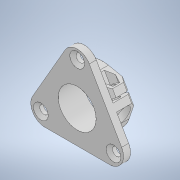
# Autodesk Inventor part: Motor Mount Insert
Saved by Autodesk Inventor 2022 (Build 260153000, 153)
## iProperties
Created: 2022-08-19
Part Number: Motor Mount Insert
Material: Generic
Document SubType Name: Modeling
Designer: Nick
Density: 1.32599 g/cm^3
Appearance: Default
Mass: 5.34 g
Surface Area: 34.9008 cm^2
Volume: 4.02719 cm^3
Author: Nick
Autodesk Inventor part; units mm, degrees
ref_plane "YZ Plane" through (0, 0, 0) normal (1, 0, 0) x (0, 1, 0)
ref_plane "XZ Plane" through (0, 0, 0) normal (0, 1, 0) x (-1, 0, 0)
ref_plane "XY Plane" through (0, 0, 0) normal (0, 0, 1) x (1, 0, 0)
sketch "Sketch1" plane through (0, 0, 0) normal (0, 0, 1) x (1, 0, 0)
  circle A0 centre (0, 16) radius 2
  circle A1 centre (-13.8564, -8) radius 2
  circle A2 centre (13.8564, -8) radius 2
  line L0 (0, 28) -> (24.2487, -14)
  line L1 (24.2487, -14) -> (-24.2487, -14)
  line L2 (-24.2487, -14) -> (0, 28)
  circle A3 centre (0, 0) radius 8.1
  line L3 (0, 16) -> (13.8564, -8) construction
  line L4 (13.8564, -8) -> (-13.8564, -8) construction
  line L5 (-13.8564, -8) -> (0, 16) construction
  dimension "d0" = 16.2
  dimension "d1" = 4
  dimension "d2" = 4
  dimension "d3" = 4
  dimension "d4" = 16
  dimension "d5" = 6
  constraints: 12 end point, 6 coincident, 4 centre point, 2 horizontal, 14 other
  measures "d0" diameter of A3
  measures "d1" diameter of A2
  measures "d2" diameter of A1
  measures "d3" diameter of A0
  measures "d4" distance of point (0, 0) A0.centre
  measures "d5" distance between parallel lines of L0 L3
extrude "Extrusion1" add sketch "Sketch1" along normal blind 3 contours A0 | A1 | A2 | L0 L1 L2
fillet "Fillet1" radius 6 3 edges at (0, 28, 1.5) (24.2487, -14, 1.5) (-24.2487, -14, 1.5)
sketch "Sketch2" plane through (0, 0, 0) normal (0, 0, -1) x (-1, 0, 0)
  circle A0 centre (0, 0) radius 8.1 projected
  arc A1 (13.8564, -14) -> (19.0526, -5) centre (13.8564, -8) ccw projected
  line L0 (5.1962, 19) -> (19.0526, -5) projected
  arc A2 (5.1962, 19) -> (-5.1962, 19) centre (0, 16) ccw projected
  line L1 (-19.0526, -5) -> (-5.1962, 19) projected
  arc A3 (-19.0526, -5) -> (-13.8564, -14) centre (-13.8564, -8) ccw projected
  line L2 (13.8564, -14) -> (-13.8564, -14) projected
  circle A4 centre (0, 0) radius 11.9
  line L3 (-10.5557, 5.517) -> (-10.0557, 6.383)
  line L4 (-10.0557, 6.383) -> (-6.7514, 4.4753)
  line L5 (-6.7514, 4.4753) -> (-7.2514, 3.6093)
  line L6 (-7.2514, 3.6093) -> (-10.5557, 5.517)
  line L7 (0, 0) -> (-7.0014, 4.0423) construction
  circle A5 centre (0, 0) radius 8.1 construction
  line L8 (-10.0557, 6.383) -> (-11.8744, 7.433)
  line L9 (-10.5557, 5.517) -> (-12.3744, 6.567)
  line L10 (-19.0526, -5) -> (-5.1962, 19) projected
  line L11 (-13.8744, 3.9689) -> (-11.286, -3.7732)
  line L12 (-10.3744, 10.0311) -> (-2.3753, 11.6605)
  point P0 (-10.3744, 10.0311)
  point P1 (-7.2514, 3.6093)
  point P2 (-12.3744, 6.567)
  point P3 (-13.8744, 3.9689)
  dimension "d9" = 3.8
  dimension "d10" = 1
  dimension "d11" = 3
  dimension "d12" = 3
  constraints: 18 end point, 5 perpendicular, 4 point on line, 3 point on circle, 3 tangent, 2 parallel, 1 centre point, 1 midpoint, 2 other
  measures "d10" distance between parallel lines of L6 L4
  measures "d11" distance of L9.end L11.start
  measures "d12" distance of L12.start L8.end
extrude "Extrusion2" add sketch "Sketch2" along normal blind 8 contours A0 L4 A4 L6 | L4 L8 L1 L12 A4 | A4 L11 L1 L9 L6 picked at (10.5244, -0.9233)
sketch "Sketch3" plane through (6.7514, 4.4753, -8) normal (0.5, -0.8660254, 0) x (0.8660254, 0.5, 0)
  circle A0 centre (2.9577, 4) radius 1.5
  line L0 (0.4577, 5.4434) -> (2.9577, 6.8868)
  line L1 (2.9577, 6.8868) -> (5.4577, 5.4434)
  line L2 (5.4577, 5.4434) -> (5.4577, 2.5566)
  line L3 (5.4577, 2.5566) -> (2.9577, 1.1132)
  line L4 (2.9577, 1.1132) -> (0.4577, 2.5566)
  line L5 (0.4577, 2.5566) -> (0.4577, 5.4434)
  line L6 (5.9154, 8) -> (5.9154, 0) projected
  line L7 (5.9154, 0) -> (0, 0) projected
  point P0 (-8.0846, 8)
  point P1 (5.9154, 4)
  point P2 (2.9577, 0)
  dimension "d15" = 3
  dimension "d16" = 5
  constraints: 12 end point, 2 midpoint, 1 centre point, 1 coincident, 1 horizontal alignment, 1 vertical, 1 vertical alignment, 13 other
  measures "d15" diameter of A0
  measures "d16" distance between parallel lines of L2 L5
extrude "Extrusion3" cut sketch "Sketch3" against normal blind 8.75 contours A0 | L0 L1 L2 L3 L4 L5
extrude "Extrusion4" add sketch "Sketch3" against normal blind 3
sketch "Sketch4" plane through (12.3744, 6.567, 0) normal (-0.5, 0.8660254, 0) x (0.8660254, 0.5, 0)
  circle A0 centre (-2.9577, 4) radius 3
  circle A1 centre (-2.9577, 4) radius 1.5
  line L0 (-5.9154, 0) -> (-5.9154, 8) projected
  line L1 (-5.9154, 8) -> (0, 8) projected
  line L2 (0, 0) -> (0, 8) projected
  point P0 (-14, 0)
  point P1 (-5.9154, 4)
  point P2 (-2.9577, 8)
  point P3 (0, 3.4981)
  point P4 (0, 4.5019)
  dimension "d21" = 6
  dimension "d22" = 3
  constraints: 2 centre point, 2 midpoint, 1 coincident, 1 horizontal alignment, 1 vertical alignment
  measures "d21" diameter of A0
  measures "d22" diameter of A1
extrude "Extrusion5" cut sketch "Sketch4" against normal through all contours A0 L2 | L2 A0 L0 | L0 A0 | A1
extrude "Extrusion6" add sketch "Sketch4" against normal blind 3 contours L2 A0 L0 | L0 A0 | A1
sketch "Sketch5" plane through (0, 0, 0) normal (0, 0, -1) x (-1, 0, 0)
  line L0 (8.9761, 15.5471) -> (-8.9761, -15.5471)
  line L1 (-7.2514, 3.6093) -> (-12.3744, 6.567) projected
  line L2 (8.9761, 15.5471) -> (-20.2638, 11.6993)
  line L3 (-20.2638, 11.6993) -> (-8.9761, -15.5471)
  line L4 (0, 0) -> (-20.2638, 11.6993)
  line L5 (-11.8744, 7.433) -> (-6.7514, 4.4753) projected
  constraints: 8 end point, 1 coincident, 1 midpoint, 1 parallel, 1 perpendicular
extrude "Extrusion7" cut sketch "Sketch5" along normal blind 0.3 contours L0 L4 L2
sketch "Sketch6" plane through (0, 0, 3) normal (0, 0, 1) x (1, 0, 0)
  arc A0 (-19.0526, -5) -> (-13.8564, -14) centre (-13.8564, -8) ccw projected
  line L0 (-13.8564, -14) -> (13.8564, -14) projected
  arc A1 (13.8564, -14) -> (19.0526, -5) centre (13.8564, -8) ccw projected
  line L1 (19.0526, -5) -> (5.1962, 19) projected
  arc A2 (5.1962, 19) -> (-5.1962, 19) centre (0, 16) ccw projected
  line L2 (-5.1962, 19) -> (-19.0526, -5) projected
  circle A3 centre (0, 0) radius 8.1 projected
  line L3 (0, 0) -> (0, 18) construction
  line L4 (0, 0) -> (15.5885, -9) construction
  line L5 (0, 0) -> (-15.5885, -9) construction
  dimension "d32" = 2
  dimension "d33" = 2
  dimension "d34" = 2
  constraints: 6 end point, 3 point on line
  measures "d32" distance of A0.centre L5.end
  measures "d33" distance of L4.end A1.centre
  measures "d34" distance of A2.centre L3.end
hole "Hole1" at (0, 18, 3) at (15.5885, -9, 3) at (-15.5885, -9, 3) direction (0, 0, -1) diameter 3.6 end through all countersink diameter 6.3 countersink angle 90 clearance for "Flat Head Machine Screw" size "M3" standard "Ansi Metric M Profile"
sketch "Sketch7" plane through (11.3129, 2.49, -4) normal (0.5, -0.8660254, 0) x (0, 0, 1)
  arc A0 (0.5019, -2.9577) -> (-0.5019, -2.9577) centre (0, 0) ccw projected
  line L0 (-0.5019, -2.9577) -> (0.5019, -2.9577) projected
  point P0 (4, 11.0423)
hole "Hole2" at (11.3129, 2.49, -4) direction (-0.5, 0.8660254, 0) diameter 2.9 depth 7 tip angle 118 clearance for "Flat Head Machine Screw" size "M2.5" standard "Ansi Metric M Profile"
chamfer "Chamfer3" distance 1.5 angle 45 3 edges at (11.1244, 8.7321, -0.3) (11.1244, 8.7321, -8) (13.1244, 5.2679, -8)
equation "\"d33\" = d32"
equation "\"d34\" = d32"
body "Solid1"
